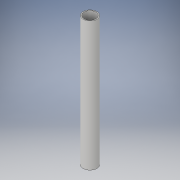
# Autodesk Inventor part: Rocket_MK_II_housing
Saved by Autodesk Inventor 2017 (Build 210142000, 142)
## iProperties
Created: 2017-05-17
Part Number: Rocket_MK_II_housing
Material: Generic
Document SubType Name: Modeling
Designer: Harrison
Density: 1 g/cm^3
Appearance: Default
Author: Harrison
Autodesk Inventor part; units mm, degrees
ref_plane "YZ Plane" through (0, 0, 0) normal (1, 0, 0) x (0, 1, 0)
ref_plane "XZ Plane" through (0, 0, 0) normal (0, 1, 0) x (-1, 0, 0)
ref_plane "XY Plane" through (0, 0, 0) normal (0, 0, 1) x (1, 0, 0)
sketch "Sketch1" plane through (0, 0, 0) normal (0, 1, 0) x (-1, 0, 0)
  circle A0 centre (0, 0) radius 13.462
  circle A1 centre (0, 0) radius 11.6078
  dimension "d0" = 26.924
  dimension "d1" = 23.2156
  constraints: 2 centre point, 2 coincident
  measures "d0" diameter of A0
  measures "d1" diameter of A1
extrude "Extrusion2" add sketch "Sketch1" along normal blind 254
body "Solid2"
